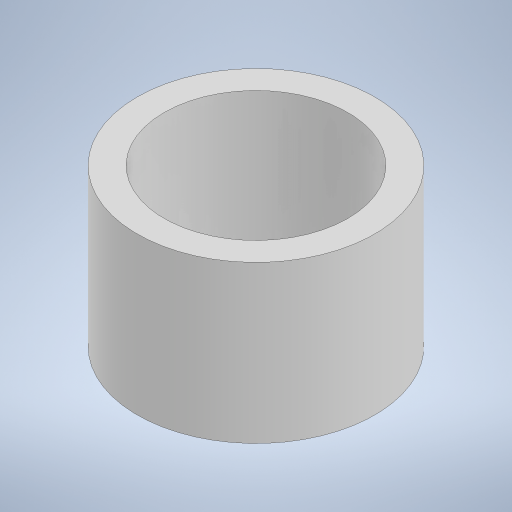
# Autodesk Inventor part: terminalcap_4.1mm
Saved by Autodesk Inventor 2023 (Build 270158000, 158)
## iProperties
Created: 2023-11-13
Part Number: terminalcap_4.1mm
Material: 일반
Document SubType Name: Modeling
Designer: Gihyeok Na
Density: 1 g/cm^3
Appearance: 기본값
Author: Gihyeok Na
Autodesk Inventor part; units mm, degrees
ref_plane "YZ Plane" through (0, 0, 0) normal (1, 0, 0) x (0, 1, 0)
ref_plane "XZ Plane" through (0, 0, 0) normal (0, 1, 0) x (-1, 0, 0)
ref_plane "XY Plane" through (0, 0, 0) normal (0, 0, 1) x (1, 0, 0)
sketch "스케치1" plane through (0, 0, 0) normal (0, 1, 0) x (-1, 0, 0)
  circle A0 centre (0, 0) radius 2.05
  circle A1 centre (0, 0) radius 2.65
  dimension "d0" = 4.1
  dimension "d1" = 5.3
  constraints: 2 centre point, 2 coincident
  measures "d0" diameter of A0
  measures "d1" diameter of A1
extrude "돌출1" add sketch "스케치1" along normal blind 3.5
